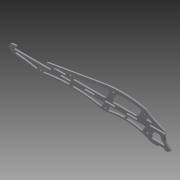
# Autodesk Inventor part: Arm_Side
Saved by Autodesk Inventor 2014 SP1 (Build 180222100, 222)
## iProperties
Created: 2014-07-26
Part Number: Arm_Side
Material: Generic
Document SubType Name: Modeling
Designer: Ryan
Density: 1 g/cm^3
Appearance: Default
Author: Ryan
Autodesk Inventor part; units mm, degrees
ref_plane "YZ Plane" through (0, 0, 0) normal (1, 0, 0) x (0, 1, 0)
ref_plane "XZ Plane" through (0, 0, 0) normal (0, 1, 0) x (-1, 0, 0)
ref_plane "XY Plane" through (0, 0, 0) normal (0, 0, 1) x (1, 0, 0)
sketch "Arm_side" plane through (0, 0, 0) normal (0, 0, 1) x (1, 0, 0)
  line L0 (8.0275, 17.0113) -> (58.3871, 17)
  arc A0 (0.004, 16.7841) -> (10.5592, 11.0108) centre (9.9939, 22.5128) ccw
  arc A1 (0, 17.2273) -> (0.004, 16.7841) centre (0.4502, 17.0097) ccw
  arc A2 (39.3008, 6.789) -> (10.5592, 11.0108) centre (-15.4059, -265.7064) ccw
  arc A3 (128.9625, 6.0746) -> (46.8779, 6.7319) centre (86.221, -205.8018) ccw
  arc A4 (39.3008, 6.789) -> (46.8779, 6.7319) centre (43.2375, 26.3977) ccw
  arc A5 (128.9625, 6.0746) -> (137.5033, 6.2125) centre (132.9174, 25.6796) ccw
  arc A6 (196.5282, 0.6084) -> (137.5033, 6.2125) centre (158.7275, -83.8856) ccw
  arc A7 (196.5282, 0.6084) -> (198.5698, 0.1725) centre (198.57, 5.1725) ccw
  line L1 (222.207, 3.7279) -> (215.3855, 10.1543)
  arc A8 (221.5213, 2) -> (222.207, 3.7279) centre (221.5213, 3) ccw
  arc A9 (214.6449, 18.6527) -> (215.3855, 10.1543) centre (223.0413, 15.103) ccw
  arc A10 (214.6449, 18.6527) -> (214.4146, 19) centre (214.4146, 18.75) ccw
  line L2 (214.3618, 0) -> (214.3618, 2)
  line L3 (214.3618, 2) -> (204.951, 2)
  line L4 (204.9482, 0.172) -> (204.951, 2)
  line L5 (214.3618, 0) -> (218.9848, 0)
  line L6 (218.9848, 0) -> (218.9848, 2)
  line L7 (218.9848, 2) -> (221.5213, 2)
  line L8 (204.9482, 0.172) -> (198.5698, 0.1725)
  line L9 (10.5257, 22.0173) -> (6.7285, 22.02)
  arc A11 (10.7256, 21.8165) -> (10.5257, 22.0173) centre (10.5256, 21.8173) ccw
  arc A12 (6.7285, 22.02) -> (0, 17.2273) centre (7.7324, 13.4911) ccw
  circle A13 centre (44.0305, 10.8938) radius 1.6
  circle A14 centre (132.9413, 10.1829) radius 1.6
  circle A15 centre (190.7645, 9.2614) radius 1.6
  line L10 (130.3716, 15.2724) -> (89.7117, 15.276)
  arc A16 (89.7117, 15.276) -> (88.8694, 14.815) centre (89.7117, 14.276) ccw
  arc A17 (131.2137, 13.7333) -> (130.3716, 15.2724) centre (130.3715, 14.2724) ccw
  line L11 (141.2939, 15.2733) -> (161.4013, 15.2733)
  arc A18 (161.8224, 14.5037) -> (161.4013, 15.2733) centre (161.4013, 14.7733) ccw
  line L12 (165.4094, 15.2733) -> (187.7253, 15.2733)
  arc A19 (165.4094, 15.2733) -> (163.7249, 14.3514) centre (165.4094, 13.2733) ccw
  arc A20 (141.2939, 15.2733) -> (139.6094, 14.3514) centre (141.2939, 13.2733) ccw
  arc A21 (188.1482, 14.5064) -> (187.7253, 15.2733) centre (187.7253, 14.7733) ccw
  line L13 (183.9824, 7.9049) -> (188.1482, 14.5064)
  line L14 (199.7163, 14.3459) -> (196.2826, 8.9425)
  arc A22 (196.2826, 8.9425) -> (198.3926, 5.1016) centre (198.3926, 7.6016) ccw
  line L15 (213.229, 5.1016) -> (198.3926, 5.1016)
  line L16 (8.0275, 17.0113) -> (8.0275, 19.1113)
  line L17 (10.726, 19.1113) -> (10.7256, 21.8165)
  line L18 (8.0275, 19.1113) -> (10.726, 19.1113)
  line L19 (58.3871, 17) -> (58.3871, 19.1)
  arc A23 (187.9852, 35.3888) -> (200.9495, 27.7571) centre (238.2867, 106.0097) ccw
  arc A24 (200.9495, 27.7571) -> (200.9628, 27.7513) centre (201.0356, 27.9376) ccw
  arc A25 (187.9852, 35.3888) -> (136.004, 37.8981) centre (154.6319, -115.8798) ccw
  line L20 (136.004, 37.8981) -> (55.0202, 23.807)
  line L21 (182.1991, 28.7895) -> (177.5147, 22.9502)
  arc A26 (173.6146, 21.079) -> (177.5147, 22.9502) centre (173.6146, 26.079) ccw
  line L22 (138.8327, 30.1246) -> (134.5524, 23.3954)
  arc A27 (130.3336, 21.079) -> (134.5524, 23.3954) centre (130.3336, 26.079) ccw
  circle A28 centre (186.6511, 28.961) radius 1
  circle A29 centre (143.7914, 34.4189) radius 1.6
  circle A30 centre (85.049, 24.8066) radius 1.6
  line L23 (191.113, 27.4048) -> (189.3001, 25.0927)
  arc A31 (189.3001, 25.0927) -> (190.087, 23.4757) centre (190.087, 24.4757) ccw
  line L24 (190.087, 23.4757) -> (196.7454, 23.4757)
  line L25 (197.034, 24.384) -> (192.4771, 27.6044)
  arc A32 (196.7454, 23.4757) -> (197.034, 24.384) centre (196.7454, 23.9757) ccw
  arc A33 (192.4771, 27.6044) -> (191.113, 27.4048) centre (191.8999, 26.7878) ccw
  line L26 (215.3065, 22.1447) -> (200.9628, 27.7513)
  arc A34 (215.1244, 21) -> (215.3065, 22.1447) centre (214.9957, 21.6073) ccw
  arc A35 (180.6693, 32.8183) -> (152.5021, 35.0076) centre (154.6319, -119.8798) ccw
  arc A36 (182.1991, 28.7895) -> (180.6693, 32.8183) centre (180.2491, 30.3538) ccw
  arc A37 (152.5021, 35.0076) -> (148.352, 32.6916) centre (152.5708, 30.0081) ccw
  line L27 (136.004, 33.8981) -> (92.1923, 26.2749)
  arc A38 (92.1923, 26.2749) -> (90.8476, 25.3779) centre (92.5351, 24.3045) ccw
  arc A39 (136.4295, 33.9491) -> (136.004, 33.8981) centre (154.6319, -119.8798) ccw
  arc A40 (138.8327, 30.1246) -> (136.4295, 33.9491) centre (136.7233, 31.4664) ccw
  arc A41 (55.0202, 23.807) -> (49.2107, 19.3981) centre (55.4654, 17.1885) ccw
  arc A42 (49.2107, 19.3981) -> (49.385, 19.1) centre (49.385, 19.3) ccw
  line L28 (58.3871, 19.1) -> (49.385, 19.1)
  line L29 (10.6063, 15.0107) -> (40.7642, 15.004)
  arc A43 (41.6062, 13.4649) -> (40.7642, 15.004) centre (40.7639, 14.004) ccw
  arc A44 (38.0241, 9.0422) -> (10.5128, 13.0151) centre (-15.4059, -263.7064) ccw
  arc A45 (38.0241, 9.0422) -> (39.0586, 9.4845) centre (38.2163, 10.0236) ccw
  arc A46 (10.6063, 15.0107) -> (10.5128, 13.0151) centre (10.6061, 14.0107) ccw
  arc A47 (82.6406, 12.313) -> (48.7884, 9.0766) centre (86.221, -203.8018) ccw
  arc A48 (82.6406, 12.313) -> (83.4663, 12.7738) centre (82.624, 13.3129) ccw
  arc A49 (47.7729, 10.6006) -> (48.7884, 9.0766) centre (48.6152, 10.0615) ccw
  line L30 (41.6062, 13.4649) -> (39.0586, 9.4845)
  line L31 (50.2948, 14.5407) -> (47.7729, 10.6006)
  line L32 (51.1372, 15.0016) -> (83.0641, 15.0004)
  arc A50 (51.1372, 15.0016) -> (50.2948, 14.5407) centre (51.137, 14.0016) ccw
  arc A51 (127.0814, 8.4454) -> (128.1127, 8.8882) centre (127.2705, 9.4273) ccw
  line L33 (139.6094, 14.3514) -> (136.6864, 9.7845)
  line L34 (131.2137, 13.7333) -> (128.1127, 8.8882)
  line L35 (88.8694, 14.815) -> (88.2598, 13.8626)
  arc A52 (182.8758, 7.4732) -> (162.2264, 10.6125) centre (158.7275, -81.8856) ccw
  arc A53 (161.8241, 11.3816) -> (162.2264, 10.6125) centre (162.2453, 11.1121) ccw
  arc A54 (158.2885, 10.6776) -> (137.7552, 8.2714) centre (158.7275, -81.8856) ccw
  arc A55 (158.2885, 10.6776) -> (159.9635, 11.5994) centre (158.279, 12.6775) ccw
  arc A56 (182.8758, 7.4732) -> (183.9824, 7.9049) centre (183.1367, 8.4386) ccw
  arc A57 (136.6864, 9.7845) -> (137.7552, 8.2714) centre (137.5286, 9.2454) ccw
  line L36 (83.9064, 13.4613) -> (83.4663, 12.7738)
  arc A58 (83.9064, 13.4613) -> (83.0641, 15.0004) centre (83.0641, 14.0004) ccw
  arc A59 (127.0814, 8.4454) -> (89.0888, 12.3236) centre (86.221, -203.8018) ccw
  arc A60 (88.2598, 13.8626) -> (89.0888, 12.3236) centre (89.1021, 13.3236) ccw
  line L37 (77.5175, 21.0991) -> (62.4893, 21.0991)
  line L38 (79.302, 25.032) -> (62.4036, 22.0917)
  arc A61 (79.8096, 24.2711) -> (79.302, 25.032) centre (79.3877, 24.5394) ccw
  arc A62 (62.4036, 22.0917) -> (62.4893, 21.0991) centre (62.4893, 21.5991) ccw
  line L39 (79.8096, 24.2711) -> (77.9393, 21.3308)
  arc A63 (77.5175, 21.0991) -> (77.9393, 21.3308) centre (77.5175, 21.5991) ccw
  line L40 (130.3336, 21.079) -> (89.9343, 21.079)
  line L41 (173.6146, 21.079) -> (144.6079, 21.079)
  line L42 (148.352, 32.6916) -> (142.9203, 24.1524)
  arc A64 (142.9203, 24.1524) -> (144.6079, 21.079) centre (144.6079, 23.079) ccw
  line L43 (90.8476, 25.3779) -> (89.0905, 22.6157)
  arc A65 (89.0905, 22.6157) -> (89.9343, 21.079) centre (89.9343, 22.079) ccw
  line L44 (193.5177, 21) -> (215.1244, 21)
  line L45 (71.2578, 17) -> (71.2578, 19)
  line L46 (71.2578, 19) -> (85.5749, 19)
  line L47 (85.5749, 19) -> (85.5749, 17)
  line L48 (103.7603, 17) -> (103.7603, 19)
  line L49 (103.7603, 19) -> (118.268, 19)
  line L50 (118.268, 19) -> (118.268, 17)
  line L51 (131.8329, 17) -> (131.8329, 19)
  line L52 (131.8329, 19) -> (146.5785, 19)
  line L53 (146.5785, 19) -> (146.5785, 17)
  line L54 (161.7281, 17) -> (161.7281, 19)
  line L55 (161.7281, 19) -> (176.6358, 19)
  line L56 (176.6358, 19) -> (176.6358, 17)
  line L57 (71.2578, 17) -> (85.5749, 17)
  line L58 (103.7603, 17) -> (118.268, 17)
  line L59 (131.8329, 17) -> (146.5785, 17)
  line L60 (161.7281, 17) -> (176.6358, 17)
  line L61 (193.5177, 19) -> (214.4146, 19)
  line L62 (193.5177, 19) -> (193.5177, 21)
  line L63 (213.9147, 6.8295) -> (210.3855, 10.1543)
  arc A66 (213.229, 5.1016) -> (213.9147, 6.8295) centre (213.229, 6.1016) ccw
  arc A67 (209.0497, 13.6025) -> (210.3855, 10.1543) centre (218.0413, 15.103) ccw
  arc A68 (209.0497, 13.6025) -> (207.077, 15.2733) centre (207.077, 13.2733) ccw
  line L64 (201.4043, 15.2733) -> (207.077, 15.2733)
  arc A69 (201.4043, 15.2733) -> (199.7163, 14.3459) centre (201.4043, 13.2733) ccw
  line L65 (163.7249, 14.3514) -> (161.8241, 11.3816)
  line L66 (161.8224, 14.5037) -> (159.9635, 11.5994)
  point P0 (128.9436, 13.6034)
sketch "Sketch1" plane through (0, 0, 0) normal (0, 0, 1) x (1, 0, 0)
  line L0 (71.2578, 19) -> (85.5749, 19)
  line L1 (85.5749, 19) -> (85.5749, 17)
  line L2 (85.5749, 17) -> (71.2578, 17)
  line L3 (71.2578, 17) -> (71.2578, 19)
  line L4 (103.7603, 19) -> (118.268, 19)
  line L5 (118.268, 19) -> (118.268, 17)
  line L6 (118.268, 17) -> (103.7603, 17)
  line L7 (103.7603, 17) -> (103.7603, 19)
  line L8 (131.8329, 19) -> (146.5785, 19)
  line L9 (146.5785, 19) -> (146.5785, 17)
  line L10 (146.5785, 17) -> (131.8329, 17)
  line L11 (131.8329, 17) -> (131.8329, 19)
  line L12 (161.7281, 19) -> (176.6358, 19)
  line L13 (176.6358, 19) -> (176.6358, 17)
  line L14 (176.6358, 17) -> (161.7281, 17)
  line L15 (161.7281, 17) -> (161.7281, 19)
  circle A0 centre (44.0305, 10.8938) radius 1.6
  circle A1 centre (85.049, 24.8066) radius 1.6
  circle A2 centre (132.9413, 10.1829) radius 1.6
  circle A3 centre (143.7914, 34.4189) radius 1.6
  circle A4 centre (186.6511, 28.961) radius 1
  circle A5 centre (190.7645, 9.2614) radius 1.6
  arc A6 (213.229, 5.1016) -> (213.9147, 6.8295) centre (213.229, 6.1016) ccw
  arc A7 (196.2826, 8.9425) -> (198.3926, 5.1016) centre (198.3926, 7.6016) ccw
  arc A8 (201.4043, 15.2733) -> (199.7163, 14.3459) centre (201.4043, 13.2733) ccw
  arc A9 (209.0497, 13.6025) -> (207.077, 15.2733) centre (207.077, 13.2733) ccw
  line L16 (198.5698, 0.1725) -> (204.9482, 0.172)
  line L17 (204.9482, 0.172) -> (204.951, 2)
  line L18 (204.951, 2) -> (214.3618, 2)
  line L19 (214.3618, 2) -> (214.3618, 0)
  line L20 (214.3618, 0) -> (218.9848, 0)
  line L21 (218.9848, 0) -> (218.9848, 2)
  line L22 (218.9848, 2) -> (221.5213, 2)
  arc A10 (196.5282, 0.6084) -> (198.5698, 0.1725) centre (198.57, 5.1725) ccw
  arc A11 (209.0497, 13.6025) -> (210.3855, 10.1543) centre (218.0413, 15.103) ccw
  arc A12 (221.5213, 2) -> (222.207, 3.7279) centre (221.5213, 3) ccw
  arc A13 (214.6449, 18.6527) -> (215.3855, 10.1543) centre (223.0413, 15.103) ccw
  arc A14 (214.6449, 18.6527) -> (214.4146, 19) centre (214.4146, 18.75) ccw
  line L23 (215.3855, 10.1543) -> (222.207, 3.7279)
  line L24 (213.9147, 6.8295) -> (210.3855, 10.1543)
  line L25 (207.077, 15.2733) -> (201.4043, 15.2733)
  line L26 (199.7163, 14.3459) -> (196.2826, 8.9425)
  line L27 (198.3926, 5.1016) -> (213.229, 5.1016)
  arc A15 (215.1244, 21) -> (215.3065, 22.1447) centre (214.9957, 21.6073) ccw
  line L28 (193.5177, 19) -> (193.5177, 21)
  line L29 (193.5177, 21) -> (215.1244, 21)
  line L30 (214.4146, 19) -> (193.5177, 19)
  line L31 (200.9628, 27.7513) -> (215.3065, 22.1447)
  arc A16 (187.9852, 35.3888) -> (200.9495, 27.7571) centre (238.2867, 106.0097) ccw
  arc A17 (189.3001, 25.0927) -> (190.087, 23.4757) centre (190.087, 24.4757) ccw
  arc A18 (192.4771, 27.6044) -> (191.113, 27.4048) centre (191.8999, 26.7878) ccw
  arc A19 (196.7454, 23.4757) -> (197.034, 24.384) centre (196.7454, 23.9757) ccw
  line L32 (197.034, 24.384) -> (192.4771, 27.6044)
  line L33 (189.3001, 25.0927) -> (191.113, 27.4048)
  line L34 (190.087, 23.4757) -> (196.7454, 23.4757)
  arc A20 (165.4094, 15.2733) -> (163.7249, 14.3514) centre (165.4094, 13.2733) ccw
  arc A21 (161.8241, 11.3816) -> (162.2264, 10.6125) centre (162.2453, 11.1121) ccw
  arc A22 (182.8758, 7.4732) -> (183.9824, 7.9049) centre (183.1367, 8.4386) ccw
  arc A23 (188.1482, 14.5064) -> (187.7253, 15.2733) centre (187.7253, 14.7733) ccw
  arc A24 (136.6864, 9.7845) -> (137.7552, 8.2714) centre (137.5286, 9.2454) ccw
  arc A25 (141.2939, 15.2733) -> (139.6094, 14.3514) centre (141.2939, 13.2733) ccw
  arc A26 (161.8224, 14.5037) -> (161.4013, 15.2733) centre (161.4013, 14.7733) ccw
  arc A27 (158.2885, 10.6776) -> (159.9635, 11.5994) centre (158.279, 12.6775) ccw
  arc A28 (182.8758, 7.4732) -> (162.2264, 10.6125) centre (158.7275, -81.8856) ccw
  arc A29 (158.2885, 10.6776) -> (137.7552, 8.2714) centre (158.7275, -81.8856) ccw
  line L35 (136.6864, 9.7845) -> (139.6094, 14.3514)
  line L36 (141.2939, 15.2733) -> (161.4013, 15.2733)
  line L37 (159.9635, 11.5994) -> (161.8224, 14.5037)
  line L38 (163.7249, 14.3514) -> (161.8241, 11.3816)
  line L39 (183.9824, 7.9049) -> (188.1482, 14.5064)
  line L40 (187.7253, 15.2733) -> (165.4094, 15.2733)
  arc A30 (173.6146, 21.079) -> (177.5147, 22.9502) centre (173.6146, 26.079) ccw
  arc A31 (182.1991, 28.7895) -> (180.6693, 32.8183) centre (180.2491, 30.3538) ccw
  arc A32 (152.5021, 35.0076) -> (148.352, 32.6916) centre (152.5708, 30.0081) ccw
  arc A33 (142.9203, 24.1524) -> (144.6079, 21.079) centre (144.6079, 23.079) ccw
  arc A34 (180.6693, 32.8183) -> (152.5021, 35.0076) centre (154.6319, -119.8798) ccw
  line L41 (177.5147, 22.9502) -> (182.1991, 28.7895)
  line L42 (142.9203, 24.1524) -> (148.352, 32.6916)
  line L43 (144.6079, 21.079) -> (173.6146, 21.079)
  arc A35 (196.5282, 0.6084) -> (137.5033, 6.2125) centre (158.7275, -83.8856) ccw
  arc A36 (128.9625, 6.0746) -> (46.8779, 6.7319) centre (86.221, -205.8018) ccw
  arc A37 (82.6406, 12.313) -> (48.7884, 9.0766) centre (86.221, -203.8018) ccw
  arc A38 (127.0814, 8.4454) -> (89.0888, 12.3236) centre (86.221, -203.8018) ccw
  arc A39 (128.9625, 6.0746) -> (137.5033, 6.2125) centre (132.9174, 25.6796) ccw
  arc A40 (47.7729, 10.6006) -> (48.7884, 9.0766) centre (48.6152, 10.0615) ccw
  arc A41 (127.0814, 8.4454) -> (128.1127, 8.8882) centre (127.2705, 9.4273) ccw
  arc A42 (131.2137, 13.7333) -> (130.3716, 15.2724) centre (130.3715, 14.2724) ccw
  line L44 (47.7729, 10.6006) -> (50.2948, 14.5407)
  line L45 (51.1372, 15.0016) -> (83.0641, 15.0004)
  line L46 (83.4663, 12.7738) -> (83.9064, 13.4613)
  arc A43 (82.6406, 12.313) -> (83.4663, 12.7738) centre (82.624, 13.3129) ccw
  arc A44 (83.9064, 13.4613) -> (83.0641, 15.0004) centre (83.0641, 14.0004) ccw
  arc A45 (51.1372, 15.0016) -> (50.2948, 14.5407) centre (51.137, 14.0016) ccw
  line L47 (89.7117, 15.276) -> (130.3716, 15.2724)
  line L48 (128.1127, 8.8882) -> (131.2137, 13.7333)
  line L49 (88.2598, 13.8626) -> (88.8694, 14.815)
  arc A46 (89.7117, 15.276) -> (88.8694, 14.815) centre (89.7117, 14.276) ccw
  arc A47 (88.2598, 13.8626) -> (89.0888, 12.3236) centre (89.1021, 13.3236) ccw
  arc A48 (39.3008, 6.789) -> (46.8779, 6.7319) centre (43.2375, 26.3977) ccw
  arc A49 (39.3008, 6.789) -> (10.7275, 11.0255) centre (-15.4059, -263.7064) ccw
  arc A50 (0, 17.2273) -> (0.0618, 16.6948) centre (0.4502, 17.0097) ccw
  arc A51 (-0.0169, 16.8314) -> (10.7275, 11.0255) centre (9.9939, 22.5128) ccw
  arc A52 (6.7285, 22.02) -> (0, 17.2273) centre (7.7324, 13.4911) ccw
  arc A53 (10.7256, 21.8173) -> (10.5257, 22.0173) centre (10.5256, 21.8173) ccw
  line L50 (6.7285, 22.02) -> (10.5257, 22.0173)
  line L51 (10.726, 19.1113) -> (10.7256, 21.8173)
  line L52 (10.726, 19.1113) -> (8.0275, 19.1113)
  line L53 (8.0275, 19.1113) -> (8.027, 17.0113)
  line L54 (8.027, 17.0113) -> (58.3871, 17)
  line L55 (58.3871, 17) -> (58.3871, 19.1)
  arc A54 (41.6062, 13.4649) -> (40.7642, 15.004) centre (40.7639, 14.004) ccw
  arc A55 (38.0241, 9.0422) -> (39.0586, 9.4845) centre (38.2163, 10.0236) ccw
  arc A56 (10.6063, 15.0107) -> (10.5128, 13.0151) centre (10.6061, 14.0107) ccw
  arc A57 (38.0241, 9.0422) -> (10.5128, 13.0151) centre (-15.4059, -263.7064) ccw
  line L56 (40.7642, 15.004) -> (10.6063, 15.0107)
  line L57 (39.0586, 9.4845) -> (41.6062, 13.4649)
  arc A58 (49.2107, 19.3981) -> (49.385, 19.1) centre (49.385, 19.3) ccw
  line L58 (49.385, 19.1) -> (58.3871, 19.1)
  arc A59 (55.0202, 23.807) -> (49.2107, 19.3981) centre (55.4654, 17.1885) ccw
  line L59 (136.004, 37.8981) -> (55.0202, 23.807)
  arc A60 (187.9852, 35.3888) -> (136.004, 37.8981) centre (154.6319, -115.8798) ccw
  arc A61 (77.5175, 21.0991) -> (77.9393, 21.3308) centre (77.5175, 21.5991) ccw
  arc A62 (79.8096, 24.2711) -> (79.302, 25.032) centre (79.3877, 24.5394) ccw
  arc A63 (62.4036, 22.0917) -> (62.4893, 21.0991) centre (62.4893, 21.5991) ccw
  line L60 (62.4036, 22.0917) -> (79.302, 25.032)
  line L61 (77.9393, 21.3308) -> (79.8096, 24.2711)
  line L62 (77.5175, 21.0991) -> (62.4893, 21.0991)
  arc A64 (138.8327, 30.1246) -> (136.4295, 33.9491) centre (136.7233, 31.4664) ccw
  arc A65 (130.3336, 21.079) -> (134.5524, 23.3954) centre (130.3336, 26.079) ccw
  arc A66 (89.0905, 22.6157) -> (89.9343, 21.079) centre (89.9343, 22.079) ccw
  arc A67 (92.1923, 26.2749) -> (90.8476, 25.3779) centre (92.5351, 24.3045) ccw
  line L63 (134.5524, 23.3954) -> (138.8327, 30.1246)
  line L64 (130.3336, 21.079) -> (89.9343, 21.079)
  line L65 (90.8476, 25.3779) -> (89.0905, 22.6157)
  line L66 (92.1923, 26.2749) -> (136.4256, 33.9715)
  arc A68 (200.9495, 27.7571) -> (200.9628, 27.7513) centre (201.0356, 27.9376) ccw
  arc A69 (83.9064, 13.4613) -> (83.0641, 15.0004) centre (83.0641, 14.0004) ccw
  arc A70 (82.6406, 12.313) -> (83.4663, 12.7738) centre (82.624, 13.3129) ccw
  line L67 (83.4663, 12.7738) -> (83.9064, 13.4613)
  line L68 (83.0641, 15.0004) -> (51.1372, 15.0016)
  arc A71 (82.6406, 12.313) -> (48.7884, 9.0766) centre (86.221, -203.8018) ccw
  arc A72 (47.7729, 10.6006) -> (48.7884, 9.0766) centre (48.6152, 10.0615) ccw
  line L69 (47.7729, 10.6006) -> (50.2948, 14.5407)
  arc A73 (89.0905, 22.6157) -> (89.9343, 21.079) centre (89.9343, 22.079) ccw
  arc A74 (92.1923, 26.2749) -> (90.8476, 25.3779) centre (92.5351, 24.3045) ccw
  line L70 (89.0905, 22.6157) -> (90.8476, 25.3779)
  line L71 (92.1923, 26.2749) -> (136.4295, 33.9491)
  line L72 (130.3336, 21.079) -> (89.9343, 21.079)
  line L73 (134.5524, 23.3954) -> (138.8327, 30.1246)
  arc A75 (138.8327, 30.1246) -> (136.4295, 33.9491) centre (136.7233, 31.4664) ccw
  arc A76 (130.3336, 21.079) -> (134.5524, 23.3954) centre (130.3336, 26.079) ccw
  line L74 (8.0275, 17.0113) -> (58.3871, 17)
  arc A77 (0.004, 16.7841) -> (10.5592, 11.0108) centre (9.9939, 22.5128) ccw
  arc A78 (0, 17.2273) -> (0.004, 16.7841) centre (0.4502, 17.0097) ccw
  arc A79 (39.3008, 6.789) -> (10.5592, 11.0108) centre (-15.4059, -265.7064) ccw
  arc A80 (128.9625, 6.0746) -> (46.8779, 6.7319) centre (86.221, -205.8018) ccw
  arc A81 (39.3008, 6.789) -> (46.8779, 6.7319) centre (43.2375, 26.3977) ccw
  arc A82 (128.9625, 6.0746) -> (137.5033, 6.2125) centre (132.9174, 25.6796) ccw
  arc A83 (196.5282, 0.6084) -> (137.5033, 6.2125) centre (158.7275, -83.8856) ccw
  arc A84 (196.5282, 0.6084) -> (198.5698, 0.1725) centre (198.57, 5.1725) ccw
  line L75 (222.207, 3.7279) -> (215.3855, 10.1543)
  arc A85 (221.5213, 2) -> (222.207, 3.7279) centre (221.5213, 3) ccw
  arc A86 (214.6449, 18.6527) -> (215.3855, 10.1543) centre (223.0413, 15.103) ccw
  arc A87 (214.6449, 18.6527) -> (214.4146, 19) centre (214.4146, 18.75) ccw
  line L76 (214.3618, 0) -> (214.3618, 2)
  line L77 (214.3618, 2) -> (204.951, 2)
  line L78 (204.9482, 0.172) -> (204.951, 2)
  line L79 (214.3618, 0) -> (218.9848, 0)
  line L80 (218.9848, 0) -> (218.9848, 2)
  line L81 (218.9848, 2) -> (221.5213, 2)
  line L82 (204.9482, 0.172) -> (198.5698, 0.1725)
  line L83 (10.5257, 22.0173) -> (6.7285, 22.02)
  arc A88 (10.7256, 21.8165) -> (10.5257, 22.0173) centre (10.5256, 21.8173) ccw
  arc A89 (6.7285, 22.02) -> (0, 17.2273) centre (7.7324, 13.4911) ccw
  circle A90 centre (44.0305, 10.8938) radius 1.6
  circle A91 centre (132.9413, 10.1829) radius 1.6
  circle A92 centre (190.7645, 9.2614) radius 1.6
  line L84 (130.3716, 15.2724) -> (89.7117, 15.276)
  arc A93 (89.7117, 15.276) -> (88.8694, 14.815) centre (89.7117, 14.276) ccw
  arc A94 (131.2137, 13.7333) -> (130.3716, 15.2724) centre (130.3715, 14.2724) ccw
  line L85 (141.2939, 15.2733) -> (161.4013, 15.2733)
  arc A95 (161.8224, 14.5037) -> (161.4013, 15.2733) centre (161.4013, 14.7733) ccw
  line L86 (165.4094, 15.2733) -> (187.7253, 15.2733)
  arc A96 (165.4094, 15.2733) -> (163.7249, 14.3514) centre (165.4094, 13.2733) ccw
  arc A97 (141.2939, 15.2733) -> (139.6094, 14.3514) centre (141.2939, 13.2733) ccw
  arc A98 (188.1482, 14.5064) -> (187.7253, 15.2733) centre (187.7253, 14.7733) ccw
  line L87 (183.9824, 7.9049) -> (188.1482, 14.5064)
  line L88 (199.7163, 14.3459) -> (196.2826, 8.9425)
  arc A99 (196.2826, 8.9425) -> (198.3926, 5.1016) centre (198.3926, 7.6016) ccw
  line L89 (213.229, 5.1016) -> (198.3926, 5.1016)
  line L90 (8.0275, 17.0113) -> (8.0275, 19.1113)
  line L91 (10.726, 19.1113) -> (10.7256, 21.8165)
  line L92 (8.0275, 19.1113) -> (10.726, 19.1113)
  line L93 (58.3871, 17) -> (58.3871, 19.1)
  arc A100 (187.9852, 35.3888) -> (200.9495, 27.7571) centre (238.2867, 106.0097) ccw
  arc A101 (200.9495, 27.7571) -> (200.9628, 27.7513) centre (201.0356, 27.9376) ccw
  arc A102 (187.9852, 35.3888) -> (136.004, 37.8981) centre (154.6319, -115.8798) ccw
  line L94 (136.004, 37.8981) -> (55.0202, 23.807)
  line L95 (182.1991, 28.7895) -> (177.5147, 22.9502)
  arc A103 (173.6146, 21.079) -> (177.5147, 22.9502) centre (173.6146, 26.079) ccw
  line L96 (138.8327, 30.1246) -> (134.5524, 23.3954)
  arc A104 (130.3336, 21.079) -> (134.5524, 23.3954) centre (130.3336, 26.079) ccw
  circle A105 centre (186.6511, 28.961) radius 1
  circle A106 centre (143.7914, 34.4189) radius 1.6
  circle A107 centre (85.049, 24.8066) radius 1.6
  line L97 (191.113, 27.4048) -> (189.3001, 25.0927)
  arc A108 (189.3001, 25.0927) -> (190.087, 23.4757) centre (190.087, 24.4757) ccw
  line L98 (190.087, 23.4757) -> (196.7454, 23.4757)
  line L99 (197.034, 24.384) -> (192.4771, 27.6044)
  arc A109 (196.7454, 23.4757) -> (197.034, 24.384) centre (196.7454, 23.9757) ccw
  arc A110 (192.4771, 27.6044) -> (191.113, 27.4048) centre (191.8999, 26.7878) ccw
  line L100 (215.3065, 22.1447) -> (200.9628, 27.7513)
  arc A111 (215.1244, 21) -> (215.3065, 22.1447) centre (214.9957, 21.6073) ccw
  arc A112 (180.6693, 32.8183) -> (152.5021, 35.0076) centre (154.6319, -119.8798) ccw
  arc A113 (182.1991, 28.7895) -> (180.6693, 32.8183) centre (180.2491, 30.3538) ccw
  arc A114 (152.5021, 35.0076) -> (148.352, 32.6916) centre (152.5708, 30.0081) ccw
  line L101 (136.004, 33.8981) -> (92.1923, 26.2749)
  arc A115 (92.1923, 26.2749) -> (90.8476, 25.3779) centre (92.5351, 24.3045) ccw
  arc A116 (136.4295, 33.9491) -> (136.004, 33.8981) centre (154.6319, -119.8798) ccw
  arc A117 (138.8327, 30.1246) -> (136.4295, 33.9491) centre (136.7233, 31.4664) ccw
  arc A118 (55.0202, 23.807) -> (49.2107, 19.3981) centre (55.4654, 17.1885) ccw
  arc A119 (49.2107, 19.3981) -> (49.385, 19.1) centre (49.385, 19.3) ccw
  line L102 (58.3871, 19.1) -> (49.385, 19.1)
  line L103 (10.6063, 15.0107) -> (40.7642, 15.004)
  arc A120 (41.6062, 13.4649) -> (40.7642, 15.004) centre (40.7639, 14.004) ccw
  arc A121 (38.0241, 9.0422) -> (10.5128, 13.0151) centre (-15.4059, -263.7064) ccw
  arc A122 (38.0241, 9.0422) -> (39.0586, 9.4845) centre (38.2163, 10.0236) ccw
  arc A123 (10.6063, 15.0107) -> (10.5128, 13.0151) centre (10.6061, 14.0107) ccw
  arc A124 (82.6406, 12.313) -> (48.7884, 9.0766) centre (86.221, -203.8018) ccw
  arc A125 (82.6406, 12.313) -> (83.4663, 12.7738) centre (82.624, 13.3129) ccw
  arc A126 (47.7729, 10.6006) -> (48.7884, 9.0766) centre (48.6152, 10.0615) ccw
  line L104 (41.6062, 13.4649) -> (39.0586, 9.4845)
  line L105 (50.2948, 14.5407) -> (47.7729, 10.6006)
  line L106 (51.1372, 15.0016) -> (83.0641, 15.0004)
  arc A127 (51.1372, 15.0016) -> (50.2948, 14.5407) centre (51.137, 14.0016) ccw
  arc A128 (127.0814, 8.4454) -> (128.1127, 8.8882) centre (127.2705, 9.4273) ccw
  line L107 (139.6094, 14.3514) -> (136.6864, 9.7845)
  line L108 (131.2137, 13.7333) -> (128.1127, 8.8882)
  line L109 (88.8694, 14.815) -> (88.2598, 13.8626)
  arc A129 (182.8758, 7.4732) -> (162.2264, 10.6125) centre (158.7275, -81.8856) ccw
  arc A130 (161.8241, 11.3816) -> (162.2264, 10.6125) centre (162.2453, 11.1121) ccw
  arc A131 (158.2885, 10.6776) -> (137.7552, 8.2714) centre (158.7275, -81.8856) ccw
  arc A132 (158.2885, 10.6776) -> (159.9635, 11.5994) centre (158.279, 12.6775) ccw
  arc A133 (182.8758, 7.4732) -> (183.9824, 7.9049) centre (183.1367, 8.4386) ccw
  arc A134 (136.6864, 9.7845) -> (137.7552, 8.2714) centre (137.5286, 9.2454) ccw
  line L110 (83.9064, 13.4613) -> (83.4663, 12.7738)
  arc A135 (83.9064, 13.4613) -> (83.0641, 15.0004) centre (83.0641, 14.0004) ccw
  arc A136 (127.0814, 8.4454) -> (89.0888, 12.3236) centre (86.221, -203.8018) ccw
  arc A137 (88.2598, 13.8626) -> (89.0888, 12.3236) centre (89.1021, 13.3236) ccw
  line L111 (77.5175, 21.0991) -> (62.4893, 21.0991)
  line L112 (79.302, 25.032) -> (62.4036, 22.0917)
  arc A138 (79.8096, 24.2711) -> (79.302, 25.032) centre (79.3877, 24.5394) ccw
  arc A139 (62.4036, 22.0917) -> (62.4893, 21.0991) centre (62.4893, 21.5991) ccw
  line L113 (79.8096, 24.2711) -> (77.9393, 21.3308)
  arc A140 (77.5175, 21.0991) -> (77.9393, 21.3308) centre (77.5175, 21.5991) ccw
  line L114 (130.3336, 21.079) -> (89.9343, 21.079)
  line L115 (173.6146, 21.079) -> (144.6079, 21.079)
  line L116 (148.352, 32.6916) -> (142.9203, 24.1524)
  arc A141 (142.9203, 24.1524) -> (144.6079, 21.079) centre (144.6079, 23.079) ccw
  line L117 (90.8476, 25.3779) -> (89.0905, 22.6157)
  arc A142 (89.0905, 22.6157) -> (89.9343, 21.079) centre (89.9343, 22.079) ccw
  line L118 (193.5177, 21) -> (215.1244, 21)
  line L119 (71.2578, 17) -> (71.2578, 19)
  line L120 (71.2578, 19) -> (85.5749, 19)
  line L121 (85.5749, 19) -> (85.5749, 17)
  line L122 (103.7603, 17) -> (103.7603, 19)
  line L123 (103.7603, 19) -> (118.268, 19)
  line L124 (118.268, 19) -> (118.268, 17)
  line L125 (131.8329, 17) -> (131.8329, 19)
  line L126 (131.8329, 19) -> (146.5785, 19)
  line L127 (146.5785, 19) -> (146.5785, 17)
  line L128 (161.7281, 17) -> (161.7281, 19)
  line L129 (161.7281, 19) -> (176.6358, 19)
  line L130 (176.6358, 19) -> (176.6358, 17)
  line L131 (71.2578, 17) -> (85.5749, 17)
  line L132 (103.7603, 17) -> (118.268, 17)
  line L133 (131.8329, 17) -> (146.5785, 17)
  line L134 (161.7281, 17) -> (176.6358, 17)
  line L135 (193.5177, 19) -> (214.4146, 19)
  line L136 (193.5177, 19) -> (193.5177, 21)
  line L137 (213.9147, 6.8295) -> (210.3855, 10.1543)
  arc A143 (213.229, 5.1016) -> (213.9147, 6.8295) centre (213.229, 6.1016) ccw
  arc A144 (209.0497, 13.6025) -> (210.3855, 10.1543) centre (218.0413, 15.103) ccw
  arc A145 (209.0497, 13.6025) -> (207.077, 15.2733) centre (207.077, 13.2733) ccw
  line L138 (201.4043, 15.2733) -> (207.077, 15.2733)
  arc A146 (201.4043, 15.2733) -> (199.7163, 14.3459) centre (201.4043, 13.2733) ccw
  line L139 (163.7249, 14.3514) -> (161.8241, 11.3816)
  line L140 (161.8224, 14.5037) -> (159.9635, 11.5994)
  point P0 (0, 0)
  point P1 (83.0641, 15.0004)
  constraints: 148 end point, 146 point on circle, 84 tangent, 77 centre point, 33 horizontal, 8 parallel, 5 perpendicular, 3 collinear, 3 vertical, 2 concentric, 1 equal length, 1 point on line, 333 other
extrude "Extrusion1" add sketch "Sketch1" along normal blind 2 contours A10 A35 A39 A36 A48 A49 A51 A50 A52 L50 A53 L51 L52 L53 L54 L55 L58 A58 A59 L59 A60 A16 A68 L31 A15 L29 L28 L30 A14 A13 L23 A12 L22 L21 L20 L19 L18 L17 L16 | L71 L66 A116
body "Solid1"
